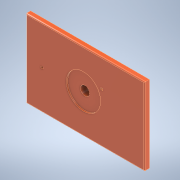
# Autodesk Inventor part: Lid
Saved by Autodesk Inventor 2022.2 (Build 262287010, 287A)
## iProperties
Created: 2022-03-17
Part Number: Lid
Material: Genérico
Document SubType Name: Modeling
Designer: mabel
Density: 1 g/cm^3
Appearance: Suave - Naranja claro
Author: mabel
Autodesk Inventor part; units mm, degrees
ref_plane "YZ Plane" through (0, 0, 0) normal (1, 0, 0) x (0, 1, 0)
ref_plane "XZ Plane" through (0, 0, 0) normal (0, 1, 0) x (-1, 0, 0)
ref_plane "XY Plane" through (0, 0, 0) normal (0, 0, 1) x (1, 0, 0)
sketch "Boceto2" plane through (0, 0, 0) normal (0, 0, 1) x (1, 0, 0)
  line L0 (130, -85) -> (-130, -85)
  line L1 (-130, -85) -> (-130, 85)
  line L2 (-130, 85) -> (130, 85)
  line L3 (130, 85) -> (130, -85)
  line L4 (130, -85) -> (-130, 85) construction
  line L5 (-130, -85) -> (130, 85) construction
  point P0 (0, 0)
  dimension "d0" = 260
  dimension "d1" = 170
  constraints: 12 end point, 2 midpoint, 2 parallel, 1 horizontal, 1 perpendicular
  measures "d0" distance of L1.end L2.end
  measures "d1" distance of L0.end L1.end
extrude "Extrusión1" add sketch "Boceto2" along normal blind 10
sketch "Boceto3" plane through (0, 0, 10) normal (0, 0, 1) x (1, 0, 0)
  line L0 (-95, 0) -> (-4.19, 0) construction
  circle A0 centre (-95, 0) radius 2.5
  circle A1 centre (-4.19, 0) radius 10
  line L1 (-130, 85) -> (-130, -85) projected
  line L2 (130, -85) -> (130, 85) projected
  line L3 (-130, -85) -> (130, -85) projected
  line L4 (130, 0) -> (80, 0) construction
  line L5 (80, 0) -> (80, -23.2237) construction
  point P0 (0, 0)
  point P1 (-130, 0)
  dimension "d7" = 5
  dimension "d8" = 20
  dimension "d14" = 85
  dimension "d29" = 50
  dimension "d30" = 90.81
  dimension "d31" = 35
  dimension "d32" = 134.19
  constraints: 6 end point, 2 centre point, 2 coincident, 2 horizontal, 2 midpoint, 1 perpendicular
  measures "d7" diameter of A0
  measures "d8" diameter of A1
  measures "d14" distance from line of L3 L0.end
  measures "d29" distance of L4.start L4.end
  measures "d30" distance of A1.centre A0.centre
  measures "d31" distance from line of A0.centre L1
  measures "d32" distance from line of L2 A1.centre
extrude "Extrusión2" cut sketch "Boceto3" against normal through all
sketch "Boceto5" plane through (0, 0, 0) normal (0, 0, -1) x (-1, 0, 0)
  line L0 (-130, -85) -> (-130, 85) projected
  line L1 (130, -85) -> (-130, -85)
  line L2 (-130, -85) -> (-130, 85)
  line L3 (-130, 85) -> (130, 85)
  line L4 (130, 85) -> (130, -85)
  line L5 (130, -85) -> (-130, 85) construction
  line L6 (-130, -85) -> (130, 85) construction
  line L7 (119.5, 74.5) -> (-119.5, 74.5)
  line L8 (-119.5, 74.5) -> (-119.5, -74.5)
  line L9 (-119.5, -74.5) -> (119.5, -74.5)
  line L10 (119.5, -74.5) -> (119.5, 74.5)
  circle A0 centre (4.19, 0) radius 10 projected
  circle A1 centre (4.19, 0) radius 20
  circle A2 centre (95, 0) radius 2.5 projected
  circle A3 centre (95, 0) radius 2.5
  point P0 (0, 0)
  dimension "d23" = 10.5
  dimension "d24" = 40
  dimension "d25" = 5
  constraints: 20 end point, 4 parallel, 2 centre point, 2 coincident, 2 midpoint, 2 perpendicular, 1 horizontal, 1 horizontal alignment, 3 other
  measures "d23" distance between parallel lines of L3 L7
  measures "d24" diameter of A1
  measures "d25" diameter of A3
extrude "Extrusión4" add sketch "Boceto5" along normal blind 10 contours L10 L9 L8 L7 | A1
fillet "Empalme1" radius 2 1 edges at (0, -85, 10)
fillet "Empalme2" radius 2 7 edges at (0, 85, 10) (-130, -84.4142, 9.4142) (-130, -85, 4) (-130, 1, 10) (130, -84.4142, 9.4142) (130, -85, 4) (130, 1, 10)
sketch "Boceto6" plane through (0, 0, 10) normal (0, 0, 1) x (1, 0, 0)
  circle A0 centre (-4.19, 0) radius 10 projected
  line L0 (-4.19, 0) -> (35.81, 0)
  line L1 (35.81, 0) -> (35.81, 25)
  line L2 (37.81, 23.5) -> (33.81, 23.5)
  line L3 (33.81, 23.5) -> (33.81, 26.5)
  line L4 (33.81, 26.5) -> (37.81, 26.5)
  line L5 (37.81, 26.5) -> (37.81, 23.5)
  line L6 (37.81, 23.5) -> (33.81, 26.5) construction
  line L7 (33.81, 23.5) -> (37.81, 26.5) construction
  point P0 (0, 0)
  dimension "d35" = 40
  dimension "d36" = 25
  dimension "d38" = 4
  dimension "d39" = 3
  constraints: 16 end point, 2 horizontal, 2 midpoint, 2 parallel, 2 perpendicular
  measures "d35" distance of L0.start L0.end
  measures "d36" distance of L0.end L1.end
  measures "d38" distance of L3.end L4.end
  measures "d39" distance of L2.end L3.end
extrude "Extrusión5" cut sketch "Boceto6" against normal blind 1.4 contours L2 L3 L4 L5
sketch "Boceto8" plane through (0, 0, 10) normal (0, 0, 1) x (1, 0, 0)
  line L0 (33.81, 23.5) -> (33.81, 26.5) projected
  line L1 (33.81, 23.5) -> (37.81, 23.5)
  line L2 (37.81, 23.5) -> (37.81, 22.5)
  line L3 (37.81, 22.5) -> (33.81, 22.5)
  line L4 (33.81, 22.5) -> (33.81, 23.5)
  point P0 (0, 0)
  dimension "d42" = 4
  dimension "d43" = 1
  constraints: 8 end point, 2 parallel, 1 horizontal, 1 perpendicular
  measures "d42" distance of L2.end L3.end
  measures "d43" distance of L1.end L2.end
extrude "Extrusión6" cut sketch "Boceto8" against normal through all
sketch "Boceto9" plane through (0, 0, 10) normal (0, 0, 1) x (1, 0, 0)
  circle A0 centre (-4.19, 0) radius 10 projected
  circle A1 centre (-4.19, 0) radius 37.5
  circle A2 centre (-4.19, 0) radius 10
  point P0 (0, 0)
  dimension "d47" = 75
  constraints: 2 centre point, 1 coincident, 1 concentric
  measures "d47" diameter of A1
extrude "Extrusión7" cut sketch "Boceto9" against normal blind 3
sketch "Boceto10" plane through (0, 0, -10) normal (0, 0, -1) x (-1, 0, 0)
  circle A0 centre (95, 0) radius 2.5 projected
  circle A1 centre (95, 0) radius 18.5
  circle A2 centre (95, 0) radius 6
  point P0 (0, 0)
  dimension "d50" = 37
  dimension "d51" = 12
  constraints: 2 centre point, 2 coincident
  measures "d50" diameter of A1
  measures "d51" diameter of A2
extrude "Extrusión8" cut sketch "Boceto10" against normal blind 10 contours A1 | A2
sketch "Boceto11" plane through (-95, 0, 0) normal (0, 0, -1) x (-1, 0, 0)
  circle A0 centre (0, 0) radius 2.5 projected
  circle A1 centre (0, 0) radius 6
  point P0 (-95, 0)
  dimension "d54" = 12
  constraints: 1 centre point, 1 coincident
  measures "d54" diameter of A1
extrude "Extrusión9" cut sketch "Boceto11" against normal blind 5
